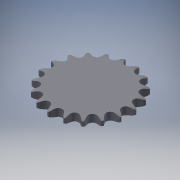
# Autodesk Inventor part: Roller Chain Sprocket2
Saved by Autodesk Inventor 2016 SP1 (Build 200210100, 210)
## iProperties
Created: 2016-01-21
Part Number: Roller Chain Sprocket2
Material: Steel
Document SubType Name: Modeling
Designer: steele
Density: 1 g/cm^3
Appearance: Steel
CustomPartVersion: 1
Author: steele
Autodesk Inventor part; units mm, degrees
ref_plane "YZ Plane" through (0, 0, 0) normal (1, 0, 0) x (0, 1, 0)
ref_plane "XZ Plane" through (0, 0, 0) normal (0, 1, 0) x (-1, 0, 0)
sketch "Theoretical Tooth Profile" plane through (0, 0, 0) normal (0, 0, 1) x (1, 0, 0)
  circle A0 centre (0, 0) radius 38.5796 construction
  line L0 (0, 0) -> (0, 38.5796) construction
  line L1 (0, 0) -> (12.5268, 36.4893) construction
  circle A1 centre (0, 0) radius 41.8635
  arc A2 (-3.1612, 36.0958) -> (3.1612, 36.0958) centre (0, 38.5796) ccw
  line L2 (0, 38.5796) -> (12.5268, 36.4893) construction
  line L3 (0, 38.5796) -> (4.9851, 42.4966) construction
  line L4 (4.9851, 42.4966) -> (-4.544, 38.431) construction
  arc A3 (6.3187, 41.3839) -> (4.924, 39.3217) centre (10.9434, 36.7535) ccw
  arc A4 (-4.924, 39.3217) -> (-6.3187, 41.3839) centre (-10.9434, 36.7535) ccw
  line L5 (-10.9434, 36.7535) -> (-4.924, 39.3217) construction
  arc A5 (-4.544, 38.431) -> (-3.1612, 36.0958) centre (4.9851, 42.4966) ccw
  line L6 (-4.544, 38.431) -> (-4.924, 39.3217)
  arc A6 (3.1612, 36.0958) -> (4.544, 38.431) centre (-4.9851, 42.4966) ccw
  line L7 (4.924, 39.3217) -> (4.544, 38.431)
  line L8 (0, 0) -> (6.8905, 41.2925) construction
  point P0 (6.2634, 37.5345)
  dimension "d0" = 77.1593
  dimension "d2" = 18.947
  dimension "d3" = 4.0203
  dimension "d10" = 128.158
  dimension "d11" = 15.053
  dimension "d12" = 6.3398
  dimension "d13" = 10.3602
  dimension "d14" = 11.0947
  dimension "d23" = 3.81
  constraints: 18 end point, 15 point on circle, 7 centre point, 3 coincident, 3 point on line, 3 symmetric about line, 3 tangent, 1 equal radius, 1 midpoint, 1 parallel, 1 vertical, 1 other
  measures "d0" diameter of A0
  measures "d2" angle of L1 L0
  measures "d3" radius of A2
  measures "d10" angle of L3 L0
  measures "d11" angle of L4 L3
  measures "d12" distance of L2.start L3.end
  measures "d13" distance of L3.end L4.end
  measures "d14" distance of A3.centre L0.end
  measures "d23" distance from line of L8.end L2
sketch "Tooth Profile" plane through (0, 0, 0) normal (0, 0, 1) x (1, 0, 0)
  circle A0 centre (0, 0) radius 41.8635 projected
  line L0 (0, 0) -> (0, 38.5796) construction
  line L1 (0, 38.5796) -> (3.7178, 37.0497) construction
  arc A1 (-3.7178, 37.0497) -> (3.7178, 37.0497) centre (0, 38.5796) ccw
  line L2 (-3.7178, 37.0497) -> (0, 38.5796) construction
  arc A2 (-3.7178, 37.0497) -> (-6.188, 41.4036) centre (-22.1856, 29.4497) ccw
  arc A3 (6.188, 41.4036) -> (3.7178, 37.0497) centre (22.1856, 29.4497) ccw
  dimension "d44" = 135.263
  dimension "d45" = 4.0203
  dimension "d46" = 19.9705
  constraints: 8 point on circle, 7 end point, 3 centre point, 2 tangent, 1 coincident, 1 equal radius, 1 symmetric about line, 1 vertical
  measures "d44" angle of L1 L2
  measures "d45" radius of A1
  measures "d46" radius of A3
sketch "Section Profile" plane through (0, 0, 0) normal (1, 0, 0) x (0, 1, 0)
  line L0 (41.8635, 0) -> (-41.8635, 0) projected
  line L1 (30.8145, 3.7612) -> (-30.8145, 3.7612)
  line L2 (-30.8145, 3.7612) -> (-30.8145, -3.7612)
  line L3 (-30.8145, -3.7612) -> (30.8145, -3.7612)
  line L4 (30.8145, -3.7612) -> (30.8145, 3.7612)
  line L5 (30.8145, 3.7612) -> (41.8635, 3.7612) construction
  line L6 (41.8635, 3.7612) -> (41.8635, -3.7612) construction
  line L7 (41.8635, -3.7612) -> (30.8145, -3.7612) construction
  line L8 (30.8145, -3.7612) -> (30.8145, 3.7612)
  arc A0 (41.8635, 2.1737) -> (35.5119, 3.7612) centre (35.5119, -9.7389) ccw
  arc A1 (35.5119, -3.7612) -> (41.8635, -2.1737) centre (35.5119, 9.7389) ccw
  line L9 (35.5119, 3.7612) -> (0, 3.7612)
  line L10 (0, 3.7612) -> (0, -3.7612)
  line L11 (0, -3.7612) -> (35.5119, -3.7612)
  line L12 (0, 3.7612) -> (0, -3.7612)
  line L13 (41.8635, 2.1737) -> (41.8635, -2.1737)
  point P0 (0, 0)
  point P1 (0, 0)
  dimension "d30" = 7.5225
  dimension "d31" = 61.6289
  dimension "d32" = 7.5225
  dimension "d33" = 1.5875
  dimension "d34" = 13.5001
  dimension "d43" = 3.7612
  constraints: 26 end point, 7 midpoint, 5 perpendicular, 4 parallel, 4 point on circle, 3 point on line, 3 symmetric about line, 2 centre point, 2 horizontal, 2 tangent, 1 collinear, 1 other
  measures "d30" distance between parallel lines of L7 L5
  measures "d31" distance between parallel lines of L2 L4
  measures "d32" distance between parallel lines of L3 L1
  measures "d33" distance from line of L13.start L5
  measures "d34" radius of A0
  measures "d43" distance between parallel lines of L3 L0
revolve "Shroud" add sketch "Section Profile" angle 360 about axis through (0, 0, 3.7612) along (0, 0, -1) contours L10 L3 L2 L0 | L0 L2 L1 L10
revolve "Strand" add sketch "Section Profile" angle 360 about axis through (0, 0, 3.7612) along (0, 0, -1) contours L13 A1 L11 L4 L0 | L0 L4 L9 A0 L13 | L4 L3 L10 L0 | L0 L10 L1 L4
pattern_of_one "Strand Pattern"
extrude "Theoretical Tooth" cut sketch "Theoretical Tooth Profile" along normal through all both and the other way through all contours A3 L7 A6 A2 A5 L6 A4 A1 picked at (0, 39.3932)
extrude "Tooth" [suppressed]
pattern_circular "Tooth Pattern" count 19 over 360 about axis through (0, 0, -10) along (0, 0, 1) of "Theoretical Tooth"
ref_plane "Timing Plane" through (0, 38.5796, 0) normal (1, 0, 0) x (0, 1, 0)
equation "\"d3\" = 0.5 * da_Dr + da_SC"
equation "\"d12\" = 0.8 * da_Dr"
equation "\"d13\" = 1.3 * da_Dr + da_SC"
equation "\"d14\" = 1.4 * da_Dr"
equation "\"d23\" = da_Ha"
equation "\"d44\" = da_Alfa"
equation "\"d45\" = da_Ri"
equation "\"d46\" = da_Re"
equation "\"d30\" = da_Bf"
equation "\"d31\" = da_Ds"
equation "\"d32\" = da_Bs"
equation "\"d33\" = da_Ba"
equation "\"d34\" = da_Rx"
equation "\"d40\" = da_pt"
equation "\"form_type\" = 0"
equation "\"da_p\" = 12.7"
equation "\"da_Dr\" = 7.9248"
equation "\"da_SC\" = 0.05791"
equation "\"da_Ha\" = 3.81"
equation "\"da_pt\" = 14.3764"
equation "\"da_Bf\" = 7.52246"
equation "\"da_Ba\" = 1.5875"
equation "\"da_Rx\" = 13.5001"
equation "\"da_Ra\" = 0.508"
equation "\"da_Bs\" = 7.52246"
equation "\"da_Ds\" = 61.62893"
equation "\"da_Re\" = 19.9705"
equation "\"da_Ri\" = 4.02031"
equation "\"da_Alfa\" = 135.263deg"
body "Solid1"
